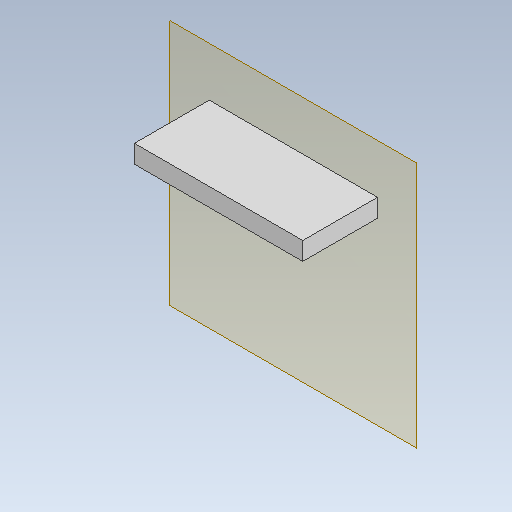
# Autodesk Inventor part: frontSupportFor-12inchBase
Saved by Autodesk Inventor 2021 (Build 250183000, 183)
## iProperties
Created: 2020-07-01
Part Number: frontSupportFor-12inchBase
Material: Generic
Document SubType Name: Modeling
Designer: robst
Density: 1 g/cm^3
Appearance: Default
Author: robst
Autodesk Inventor part; units mm, degrees
ref_plane "YZ Plane" through (0, 0, 0) normal (1, 0, 0) x (0, 1, 0)
ref_plane "XZ Plane" through (0, 0, 0) normal (0, 1, 0) x (-1, 0, 0)
ref_plane "XY Plane" through (0, 0, 0) normal (0, 0, 1) x (1, 0, 0)
ref_plane "Work Plane1" through (0, 0, 0) normal (0, 0, 1) x (1, 0, 0)
sketch "Sketch1" plane through (0, 0, 0) normal (0, 0, 1) x (1, 0, 0)
  circle A0 centre (0, 0) radius 152.4 projected
  line L0 (139.7, -76.2) -> (139.7, 76.2) projected
  line L1 (139.7, 76.2) -> (114.3, 76.2) projected
  line L2 (-114.3, 76.2) -> (-88.9, 76.2) projected
  line L3 (-88.9, 76.2) -> (-88.9, -76.2) projected
  line L4 (-114.3, 76.2) -> (114.3, 76.2)
  line L5 (114.3, 76.2) -> (114.3, 100.8031)
  line L6 (114.3, 100.8031) -> (-114.3, 100.8031)
  line L7 (-114.3, 100.8031) -> (-114.3, 76.2)
  point P0 (114.3, 76.2)
  point P1 (76.2, 76.2)
  constraints: 8 end point, 2 parallel, 1 horizontal, 1 perpendicular, 2 other
extrude "Extrusion1" add sketch "Sketch1" along normal blind 101.6 contours L5 L4 L2 L7 L6
body "Solid1"
